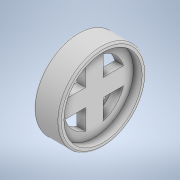
# Autodesk Inventor part: колесо
Saved by Autodesk Inventor 2020.1 (Build 241239000, 239)
## iProperties
Created: 2021-10-28
Part Number: колесо
Material: Типовые
Document SubType Name: Modeling
Designer: Ni3na
Density: 1 g/cm^3
Appearance: По умолчанию
Author: Ni3na
Autodesk Inventor part; units mm, degrees
ref_plane "YZ Plane" through (0, 0, 0) normal (1, 0, 0) x (0, 1, 0)
ref_plane "XZ Plane" through (0, 0, 0) normal (0, 1, 0) x (-1, 0, 0)
ref_plane "XY Plane" through (0, 0, 0) normal (0, 0, 1) x (1, 0, 0)
sketch "Эскиз1" plane through (0, 0, 0) normal (1, 0, 0) x (0, 1, 0)
  circle A0 centre (8.3565, 10.4457) radius 25
  point P0 (0, 0)
  dimension "d0" = 50
  constraints: 1 centre point
  measures "d0" diameter of A0
extrude "Выдавливание1" add sketch "Эскиз1" along normal blind 15
sketch "Эскиз2" plane through (0, 8.3565, 10.4457) normal (-1, 0, 0) x (0, 0, 1)
  circle A0 centre (0, 0) radius 22.5
  point P0 (-10.4457, -8.3565)
  dimension "d3" = 45
  constraints: 1 centre point
  measures "d3" diameter of A0
extrude "Выдавливание2" cut sketch "Эскиз2" against normal blind 5
sketch "Эскиз3" plane through (15, 8.3565, 10.4457) normal (1, 0, 0) x (0, 0, -1)
  circle A0 centre (0, 0) radius 22.5
  point P0 (10.4457, -8.3565)
  dimension "d6" = 45
  constraints: 1 centre point
  measures "d6" diameter of A0
extrude "Выдавливание3" cut sketch "Эскиз3" against normal blind 5
sketch "Эскиз7" plane through (5, 8.3565, 10.4457) normal (-1, 0, 0) x (0, 0, 1)
  circle A0 centre (0, 0) radius 5
  line L0 (5, 0) -> (-5, 0)
  line L1 (-5, 0) -> (-5, 30.8448)
  line L2 (-5, 30.8448) -> (5, 30.8448)
  line L3 (5, 30.8448) -> (5, 0)
  line L4 (5, 0) -> (-5, 0)
  line L5 (-5, 0) -> (-5, -27.2335)
  line L6 (-5, -27.2335) -> (5, -27.2335)
  line L7 (5, -27.2335) -> (5, 0)
  line L8 (0, -5) -> (31.8043, -5)
  line L9 (31.8043, -5) -> (31.8043, 5)
  line L10 (31.8043, 5) -> (0, 5)
  line L11 (0, 5) -> (0, -5)
  line L12 (0, -5) -> (-27.8953, -5)
  line L13 (-27.8953, -5) -> (-27.8953, 5)
  line L14 (-27.8953, 5) -> (0, 5)
  line L15 (0, 5) -> (0, -5)
  circle A1 centre (0, 0) radius 22.5
  circle A2 centre (0, 0) radius 17.5
  point P0 (-10.4457, -8.3565)
  point P1 (5, -16.7705)
  point P2 (16.7705, -5)
  point P3 (5, -5)
  point P4 (-16.7705, -5)
  point P5 (-5, -16.7705)
  point P6 (-5, -5)
  point P7 (16.7705, 5)
  point P8 (5, 16.7705)
  point P9 (5, 5)
  point P10 (-5, 16.7705)
  point P11 (-16.7705, 5)
  point P12 (-5, 5)
  dimension "d13" = 10
  dimension "d14" = 35
  constraints: 32 end point, 8 parallel, 4 horizontal, 4 perpendicular, 3 centre point, 2 coincident, 2 point on circle, 2 point on line
  measures "d13" diameter of A0
  measures "d14" diameter of A2
extrude "Выдавливание4" cut sketch "Эскиз7" against normal blind 10 contours L3 A2 L10 | L8 A2 L7 | L14 A2 L1 | L5 A2 L12
fillet "Сопряжение1" radius 1 2 edges at (15, -16.6435, 10.4457) (0, -16.6435, 10.4457)
